# Autodesk Inventor part: TPD2E001DRLR
Saved by Autodesk Inventor 2016 SP1 (Build 200210100, 210)
## iProperties
Created: 2015-11-24
Part Number: TPD2E001DRLR
Material: Generic
Document SubType Name: Modeling
Designer: PhillipD
Density: 1 g/cm^3
Appearance: TPD2E001-DRL, TPD2E001DRLR
Author: PhillipD
Autodesk Inventor part; units mm, degrees
ref_plane "YZ Plane" through (0, 0, 0) normal (1, 0, 0) x (0, 1, 0)
ref_plane "XZ Plane" through (0, 0, 0) normal (0, 1, 0) x (-1, 0, 0)
ref_plane "XY Plane" through (0, 0, 0) normal (0, 0, 1) x (1, 0, 0)
sketch "TPD2E001-DRL, TPD2E001DRLR_175" plane through (0, 0, 0) normal (0, 0, 1) x (1, 0, 0)
  line L0 (-0.9, 0.95) -> (0.9, 0.95)
  line L1 (0.9, 0.95) -> (0.9, -0.95)
  line L2 (0.9, -0.95) -> (-0.9, -0.95)
  line L3 (-0.9, -0.95) -> (-0.9, 0.95)
  constraints: 8 end point
extrude "Extrusion1" add sketch "TPD2E001-DRL, TPD2E001DRLR_175" along normal blind 1
body "Solid1"
